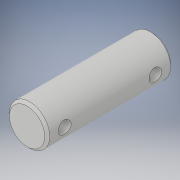
# Autodesk Inventor part: reverse gear crankshaft center rod
Saved by Autodesk Inventor 2017 (Build 210142000, 142)
## iProperties
Created: 2018-10-30
Part Number: reverse gear crankshaft center rod
Material: Generic
Document SubType Name: Modeling
Designer: User
Density: 1 g/cm^3
Appearance: Default
Author: User
Autodesk Inventor part; units mm, degrees
ref_plane "XZ Plane" through (0, 0, 0) normal (0, 1, 0) x (-1, 0, 0)
ref_plane "XY Plane" through (0, 0, 0) normal (0, 0, 1) x (1, 0, 0)
sketch "Sketch2" plane through (0, 0, 0) normal (0, 1, 0) x (-1, 0, 0)
  circle A0 centre (0, 0) radius 4
  dimension "d6" = 8
  constraints: 1 centre point, 1 coincident
  measures "d6" diameter of A0
extrude "Extrusion1" add sketch "Sketch2" along normal blind 25
chamfer "Chamfer1" distance 0.5 angle 45 1 edges at (4, 25, 0)
chamfer "Chamfer2" distance 0.5 angle 45 1 edges at (4, 0, 0)
ref_plane "Work Plane1" through (4, 0, 0) normal (1, 0, 0) x (0, 1, 0)
sketch "Sketch3" plane through (4, 0, 0) normal (1, 0, 0) x (0, 1, 0)
  circle A0 centre (3.5, 0) radius 1.25
  circle A1 centre (21.5, 0) radius 1.25
  line L0 (0, -3.5) -> (0, 3.5) construction
  line L1 (2.25, 0) -> (1.3552, 0) construction
  line L2 (22.75, 0) -> (24.5, 0) construction
  line L3 (24.5, -4) -> (24.5, 4) construction
  point P0 (0, 0)
  dimension "d15" = 2.5
  dimension "d16" = 2.5
  dimension "d17" = 18
  dimension "d19" = 3.5
  constraints: 4 end point, 2 horizontal alignment, 1 horizontal, 1 midpoint, 4 other
  measures "d17" distance of point (21.5, 0) point (3.5, 0)
  measures "d19" distance of point (0, 0) point (3.5, 0)
extrude "Extrusion2" cut sketch "Sketch3" against normal blind 25
body "Solid1"
